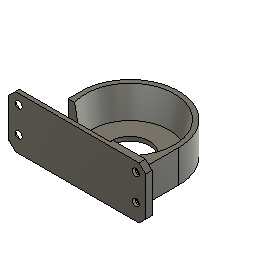
Body (Autodesk Fusion 360 design; units mm, degrees)
Autodesk Fusion 360 part; units mm, degrees
sketch "Sketch1" plane through (0, 0, 0) normal (0, 1, 0) x (1, 0, 0)
  circle A0 centre (0, 0) radius 33
  circle A1 centre (0, 0) radius 15
  circle A2 centre (0, 0) radius 37.5
  dimension "d1" = 66
  dimension "d2" = 30
  dimension "d24" = 75
  constraint coincident A0.centre A1.centre
  constraint concentric A0 A1
  constraint concentric A1 A2
  measures "d1" diameter of A0
  measures "d2" diameter of A1
  measures "d5" diameter of A0.centre
  measures "d24" diameter of A2
extrude "Extrude1" add sketch "Sketch1" along normal blind 3 contours A0 | A2 makes body 1
sketch "Sketch2" plane through (0, 3, 0) normal (0, 1, 0) x (-1, 0, 0)
  circle A0 centre (0, 0) radius 15
  circle A1 centre (0, 0) radius 33
  circle A2 centre (0, 0) radius 30
  circle A3 centre (0, 0) radius 37.5
  dimension "d5" = 60
  constraint coincident A0.centre A1.centre
  constraint concentric A1 A2
  measures "d5" diameter of A2
ref_plane "WorkPlane1" through (0, 25, 0) normal (0, 1, 0) x (-1, 0, 0)
sketch "Sketch3" plane through (0, 25, 0) normal (0, 1, 0) x (1, 0, 0)
  circle A0 centre (0, 0) radius 34
  circle A1 centre (0, 0) radius 37
  dimension "d7" = 68
  dimension "d8" = 74
  constraint coincident A0.centre A1.centre
  measures "d7" diameter of A0
  measures "d8" diameter of A1
extrude "Extrude7" add sketch "Sketch2" along normal up to surface (22 mm away) contours A1 | A3 bodies 1
loft "Loft1" add profiles "Sketch2", "Sketch3" section 1 contours A1 section 2 bodies 1
loft "Loft2" cut profiles "Sketch3", "Sketch2" section 1 contours A0 section 2 contours A2 bodies 1
sketch "Sketch9" plane through (0, 0, 0) normal (0, -1, 0) x (1, 0, 0)
  circle A0 centre (0, 0) radius 15
  circle A1 centre (0, 0) radius 37.5
  line L0 (59.9639, 0) -> (-88.3685, 0) construction
  line L1 (0, 0) -> (0, 71.4986) construction
  line L2 (37.5, 0) -> (-37.5, 0)
  line L3 (-37.5, 0) -> (-37.5, 37.5)
  line L4 (-37.5, 37.5) -> (37.5, 37.5)
  line L5 (37.5, 37.5) -> (37.5, 0)
  line L6 (37.5, 0) -> (-37.5, 37.5) construction
  line L7 (-37.5, 0) -> (37.5, 37.5) construction
  point P0 (0, 18.75)
  constraint horizontal L0
  constraint coincident A0.centre L0
  constraint coincident A0.centre A1.centre
  constraint perpendicular L0 L1
  constraint horizontal L2
  constraint perpendicular L2 L3
  constraint parallel L2 L4
  constraint parallel L3 L5
  constraint coincident L0 L2.start
  constraint coincident L6 P0
  constraint coincident L7 P0
  constraint coincident L1 P0
  constraint tangent A1 L5
  constraint tangent A1 L4
extrude "Extrude8" add sketch "Sketch9" against normal up to surface (25 mm away) contours A1 L4 L5 | A1 L3 L4 bodies 1
sketch "Sketch10" plane through (0, 0, 37.5) normal (0, 0, 1) x (1, 0, 0)
  line L0 (37.5, 25) -> (-37.5, 25)
  line L1 (-37.5, 25) -> (-37.5, 0)
  line L2 (-37.5, 0) -> (37.5, 0)
  line L3 (37.5, 0) -> (37.5, 25)
extrude "Extrude9" add sketch "Sketch10" along normal blind 3 bodies 1
sketch "Sketch12" plane through (0, 25, 0) normal (0, 1, 0) x (-1, 0, 0)
  circle A0 centre (0, 0) radius 34
  arc A1 (-37.5, 0) -> (37.5, 0) centre (0, 0) ccw
  line L0 (37.5, 0) -> (37.5, 40.5)
  line L1 (-37.5, 40.5) -> (-37.5, 0)
  line L2 (37.5, 0) -> (0.5, 0) construction
  line L3 (0.5, 0) -> (0.5, 40.5)
  line L4 (0.5, 40.5) -> (37.5, 40.5)
  line L5 (37.5, 40.5) -> (37.5, 0)
  line L6 (37.5, 40.5) -> (-37.5, 40.5)
  line L7 (37.5, 10) -> (0.5, 10)
  dimension "d52" = 10
  constraint horizontal L2
  constraint vertical L3
  constraint horizontal L4
  constraint vertical L5
  constraint coincident A1.end L0.start
  constraint collinear L4 L6
  constraint coincident L0 L7.start
  constraint coincident L3 L7.end
  constraint perpendicular L3 L7
  measures "d52" distance of L2 L7
extrude "Extrude11" cut sketch "Sketch12" against normal up to surface (22 mm away) contours A0 L3 L7 | A0 L0 L3 L4 L5 L6 L7 picked at (2.0766, 25.8639) bodies 1
ref_plane "WorkPlane2" through (0, 40, 1.5) normal (0, 1, 0) x (0, 0, 1)
sketch "Sketch14" plane through (0, 40, 1.5) normal (0, 1, 0) x (1, 0, 0)
  circle A0 centre (0, 1.5) radius 15
  circle A1 centre (0, 1.5) radius 22.5
  circle A2 centre (0, 1.5) radius 38
  dimension "d45" = 45
  dimension "d46" = 76
  constraint concentric A0 A1
  constraint concentric A0 A2
  measures "d45" diameter of A1
  measures "d46" diameter of A2
extrude "Extrude13" add sketch "Sketch14" against normal blind 3 separate body contours A2 makes body 2
sketch "Sketch16" plane through (0, 40, 0) normal (0, 1, 0) x (-1, 0, 0)
  circle A0 centre (0, 0) radius 22.5
  circle A1 centre (0, 0) radius 38
  circle A2 centre (0, 0) radius 50
  line L0 (-50, -5) -> (50, -5)
  line L1 (50, -5) -> (50, 5)
  line L2 (50, 5) -> (-50, 5)
  line L3 (-50, 5) -> (-50, -5)
  line L4 (-50, -5) -> (50, 5) construction
  line L5 (50, -5) -> (-50, 5) construction
  line L6 (-5, -50) -> (5, -50)
  line L7 (5, -50) -> (5, 50)
  line L8 (5, 50) -> (-5, 50)
  line L9 (-5, 50) -> (-5, -50)
  line L10 (-5, -50) -> (5, 50) construction
  line L11 (5, -50) -> (-5, 50) construction
  dimension "d47" = 100
  dimension "d48" = 10
  constraint concentric A0 A2
  constraint horizontal L0
  constraint perpendicular L0 L1
  constraint parallel L0 L2
  constraint parallel L1 L3
  constraint coincident L4 A0.centre
  constraint coincident L5 A0.centre
  constraint coincident A0.centre A1.centre
  constraint tangent A2 L3
  constraint horizontal L6
  constraint perpendicular L6 L7
  constraint parallel L6 L8
  constraint parallel L7 L9
  constraint coincident L10 A0.centre
  constraint coincident L11 A0.centre
  constraint equal L3 L6
  constraint tangent A2 L6
  measures "d47" diameter of A2
  measures "d48" distance of L0.start L2.end
extrude "Extrude14" add sketch "Sketch16" against normal up to surface (40 mm away) contours A1 A2 L0 L2 | A1 A2 L7 L9 | A1 A2 L0 L2 picked at (0, -41.9755) bodies 1 2
chamfer "Chamfer1" distance 12 angle 45 6 edges at (-37.6696, 38.5, -5) (-37.6696, 38.5, 5) (37.6696, 38.5, 5) (37.6696, 38.5, -5) (5, 38.5, -37.6696) (-5, 38.5, -37.6696) on bodies 2
sketch "Sketch17" plane through (0, 0, 40.5) normal (0, 0, 1) x (1, 0, 0)
  line L0 (-0.5, 3) -> (-37.5, 3)
  line L1 (-37.5, 3) -> (-37.5, 0)
  line L2 (-37.5, 0) -> (37.5, 0)
  line L3 (37.5, 0) -> (37.5, 25)
  line L4 (37.5, 25) -> (-0.5, 25)
  line L5 (-0.5, 25) -> (-0.5, 3)
  line L6 (37.5, 25) -> (52.5, 25)
  line L7 (52.5, 25) -> (52.5, 0)
  line L8 (52.5, 0) -> (37.5, 0)
  line L9 (37.5, 0) -> (37.5, 25)
  dimension "d53" = 15
  constraint horizontal L6
  constraint vertical L7
  constraint horizontal L8
  constraint vertical L9
  constraint coincident L3.end L4.start
  constraint collinear L2 L8
  measures "d53" distance of L3.end L6.end
extrude "Extrude15" add sketch "Sketch17" against normal blind 5 contours L3 L6 L7 L8 L9 bodies 1
sketch "Sketch18" plane through (0, 0, 35.5) normal (0, 0, -1) x (-1, 0, 0)
  line L0 (-52.5, 0) -> (-37.5, 0)
  line L1 (-37.5, 0) -> (-37.5, 25)
  line L2 (-37.5, 25) -> (-52.5, 25)
  line L3 (-52.5, 25) -> (-52.5, 0)
  line L4 (-37.5, 25) -> (-52.5, 0) construction
  circle A0 centre (-45, 12.5) radius 2.65
  dimension "d56" = 5.3
  constraint coincident L1.end L2.start
  constraint coincident L0.start L3.end
  constraint midpoint L4 A0.centre
  measures "d56" diameter of A0
extrude "Extrude16" cut sketch "Sketch18" against normal up to surface (5 mm away) contours A0 bodies 1
sketch "Sketch19" plane through (0, 0, 40.5) normal (0, 0, 1) x (1, 0, 0)
  line L0 (52.5, 0) -> (52.5, 25)
  line L1 (52.5, 25) -> (-0.5, 25)
  line L2 (-0.5, 25) -> (-0.5, 3)
  line L3 (-0.5, 3) -> (-37.5, 3)
  line L4 (-37.5, 3) -> (-37.5, 0)
  line L5 (-37.5, 0) -> (52.5, 0)
  circle A0 centre (45, 12.5) radius 2.65
  line L6 (52.5, 25) -> (22.5, 25)
  line L7 (22.5, 25) -> (22.5, 40)
  line L8 (22.5, 40) -> (52.5, 40)
  line L9 (52.5, 40) -> (52.5, 25)
  dimension "d61" = 15
  dimension "d62" = 30
  constraint horizontal L6
  constraint vertical L7
  constraint horizontal L8
  constraint vertical L9
  constraint collinear L0 L9
  constraint collinear L1 L6
  measures "d61" distance of L0.end L8.end
  measures "d62" distance of L7.end L8.end
extrude "Extrude17" add sketch "Sketch19" against normal blind 5 contours L1 L6 L7 L8 L9 bodies 1
sketch "Sketch20" plane through (0, 0, 35.5) normal (0, 0, -1) x (-1, 0, 0)
  circle A0 centre (-45, 12.5) radius 2.65
  line L0 (-52.5, 0) -> (-37.5, 0)
  line L1 (-37.5, 0) -> (-37.5, 25)
  line L2 (-37.5, 25) -> (-22.5, 25)
  line L3 (-22.5, 25) -> (-22.5, 40)
  line L4 (-22.5, 40) -> (-52.5, 40)
  line L5 (-52.5, 40) -> (-52.5, 0)
  line L6 (-37.5, 25) -> (-52.5, 25) construction
  line L7 (-37.5, 25) -> (-52.5, 40) construction
  circle A1 centre (-45, 32.5) radius 2.65
  constraint coincident L1.end L2.start
  constraint coincident L5 L6.end
  constraint perpendicular L5 L6
  constraint coincident L4.end L5.start
  constraint midpoint L7 A1.centre
  constraint equal A0 A1
extrude "Extrude18" cut sketch "Sketch20" against normal up to surface (5 mm away) contours A1 bodies 1
sketch "Sketch22" plane through (0, 0, 40.5) normal (0, 0, 1) x (1, 0, 0)
  circle A0 centre (45, 12.5) radius 2.65
  circle A1 centre (45, 32.5) radius 2.65
  line L0 (-0.5, 25) -> (-0.5, 3)
  line L1 (-0.5, 3) -> (-37.5, 3)
  line L2 (-37.5, 3) -> (-37.5, 0)
  line L3 (-37.5, 0) -> (52.5, 0)
  line L4 (52.5, 0) -> (52.5, 40)
  line L5 (52.5, 40) -> (22.5, 40)
  line L6 (22.5, 25) -> (-0.5, 25)
  line L7 (-52.5, 0) -> (22.5, 0)
  line L8 (22.5, 0) -> (22.5, 40)
  line L9 (22.5, 40) -> (-52.5, 40)
  line L10 (-52.5, 40) -> (-52.5, 0)
  line L11 (22.5, 40) -> (22.5, 25)
  dimension "d73" = 15
  constraint horizontal L7
  constraint vertical L8
  constraint horizontal L9
  constraint vertical L10
  constraint collinear L5 L9
  constraint coincident L5.end L8
  constraint collinear L3 L7
  measures "d73" distance of L2.end L10
extrude "Extrude19" add sketch "Sketch22" against normal blind 3 contours L0 L1 L2 L3 L6 L7 L8 | L0 L1 L2 L6 L7 L8 L9 L10 L11 bodies 1
sketch "Sketch23" plane through (0, 0, 40.5) normal (0, 0, 1) x (1, 0, 0)
  line L0 (52.5, 0) -> (52.5, 40)
  line L1 (52.5, 40) -> (-52.5, 40)
  line L2 (-52.5, 40) -> (-52.5, 0)
  line L3 (-52.5, 0) -> (52.5, 0)
  circle A0 centre (45, 32.5) radius 2.65
  circle A1 centre (45, 12.5) radius 2.65
  line L4 (45, 32.5) -> (-52.5, 32.5) construction
  line L5 (45, 12.5) -> (-52.5, 12.5) construction
  circle A2 centre (-45, 32.5) radius 2.65
  line L6 (-45, 32.5) -> (-45, 12.5) construction
  circle A3 centre (-45, 12.5) radius 2.65
  line L7 (45, 32.5) -> (52.5, 32.5)
  line L8 (-45, 32.5) -> (-52.5, 32.5)
  constraint coincident A0.centre L4.start
  constraint coincident L2 L4.end
  constraint perpendicular L2 L4
  constraint coincident A1.centre L5.start
  constraint coincident L2 L5.end
  constraint perpendicular L2 L5
  constraint coincident L4 A2.centre
  constraint coincident A2.centre L6.start
  constraint coincident L5 L6.end
  constraint perpendicular L5 L6
  constraint coincident L6.end A3.centre
  constraint equal A0 A2
  constraint equal A2 A3
  constraint coincident L0 L7.end
  constraint perpendicular L0 L7
  constraint equal L7 L8
extrude "Extrude20" cut sketch "Sketch23" against normal up to surface (3 mm away) contours A2 | A3 bodies 1
chamfer "Chamfer4" distance 5 angle 45 4 edges at (52.5, 40, 38) (52.5, 0, 38) (-52.5, 0, 39) (-52.5, 40, 39) on bodies 1
chamfer "Chamfer3" distance 15 angle 45 1 edges at (22.5, 25, 36.5) on bodies 1
chamfer "Chamfer5" distance 3 angle 45 4 edges at (47.4707, 33.4583, 35.5) (47.4707, 13.4583, 35.5) (-47.4707, 31.5417, 37.5) (-47.4707, 11.5417, 37.5) on bodies 1
sketch "Sketch24" plane through (0, 0, 0) normal (0, -1, 0) x (1, 0, 0)
  line L0 (-47.5, 40.5) -> (-47.5, 37.5)
  line L1 (-47.5, 37.5) -> (-37.5, 37.5)
  line L2 (-37.5, 37.5) -> (-37.5, 0)
  arc A0 (-37.5, 0) -> (37.5, 0) centre (0, 0) ccw
  line L3 (37.5, 0) -> (37.5, 35.5)
  line L4 (37.5, 35.5) -> (47.5, 35.5)
  line L5 (47.5, 35.5) -> (47.5, 40.5)
  line L6 (47.5, 40.5) -> (-47.5, 40.5)
  circle A1 centre (0, 0) radius 15
  circle A2 centre (0, 0) radius 17.5
  circle A3 centre (0, 0) radius 50.635
  dimension "d76" = 35
  constraint concentric A0 A2
  constraint concentric A0 A3
  measures "d76" diameter of A2
extrude "Extrude21" add sketch "Sketch24" along normal blind 3 separate body contours L2 A0 L3 L6 A3 | L2 A0 L3 A3 | A2 makes body 3
extrude "Extrude22" add sketch "Sketch24" along normal blind 45 contours A2 bodies 3
hidden bodies 2 3
